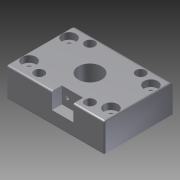
# Autodesk Inventor part: V5 Z Top bearing
Saved by Autodesk Inventor 2012 (Build 160160000, 160)
## iProperties
Created: 2013-02-06
Part Number: V5 Z Top bearing
Material: Default
Document SubType Name: Modeling
Designer: mce
Density: 1 g/cm^3
Mass: 38.3843 g
Surface Area: 115.42 cm^2
Volume: 38.3843 cm^3
Author: mce
Autodesk Inventor part; units mm, degrees
ref_plane "YZ Plane" through (0, 0, 0) normal (1, 0, 0) x (0, 1, 0)
ref_plane "XZ Plane" through (0, 0, 0) normal (0, 1, 0) x (-1, 0, 0)
ref_plane "XY Plane" through (0, 0, 0) normal (0, 0, 1) x (1, 0, 0)
sketch "Sketch1" plane through (0, 0, 0) normal (0, 0, 1) x (1, 0, 0)
  line L0 (0, 0) -> (60, 0)
  line L1 (60, 0) -> (60, 42.4)
  line L2 (60, 42.4) -> (0, 42.4)
  line L3 (0, 42.4) -> (0, 0)
  circle A0 centre (5, 33.4) radius 2.1
  circle A1 centre (55, 33.4) radius 2.1
  circle A2 centre (55, 9) radius 2.1
  circle A3 centre (5, 9) radius 2.1
  circle A4 centre (30, 21.2) radius 5
  circle A5 centre (14.5, 36.7) radius 3
  circle A6 centre (45.5, 36.7) radius 3
  circle A7 centre (45.5, 5.7) radius 3
  circle A8 centre (14.5, 5.7) radius 3
  dimension "d0" = 42.4
  dimension "d1" = 60
  dimension "d2" = 10
  dimension "d3" = 4.2
  dimension "d4" = 24.4
  dimension "d5" = 50
  dimension "d6" = 9
  dimension "d7" = 5
  dimension "d8" = 6
  dimension "d9" = 31
  dimension "d10" = 31
  dimension "d11" = 5.7
  dimension "d12" = 14.5
  dimension "d13" = 30
  dimension "d14" = 21.2
  constraints: 9 centre point, 8 end point, 6 equal radius, 4 horizontal alignment, 4 vertical alignment, 2 horizontal, 2 vertical
  measures "d0" distance of L2.end L0.start
  measures "d1" distance of L0.start L0.end
  measures "d2" diameter of A4
  measures "d3" diameter of A0
  measures "d4" distance of A3.centre A0.centre
  measures "d5" distance of A0.centre A1.centre
  measures "d6" distance from line of L2 A0.centre
  measures "d7" distance from line of L3 A0.centre
  measures "d8" diameter of A5
  measures "d9" distance of A6.centre A5.centre
  measures "d10" distance of A8.centre A5.centre
  measures "d11" distance from line of L0 A7.centre
  measures "d12" distance from line of L3 A8.centre
  measures "d13" distance from line of L3 A4.centre
  measures "d14" distance from line of L0 A4.centre
extrude "Extrusion1" add sketch "Sketch1" along normal blind 18
fillet "Fillet1" radius 1 11 edges at (0, 42.4, 9) (60, 42.4, 9) (30, 42.4, 0) (60, 21.2, 18) (30, 0, 18) (0, 21.2, 18) (0, 0, 9) (0, 21.2, 0) (60, 0, 9) (60, 21.2, 0) (30, 0, 0)
fillet "Fillet2" radius 3 3 edges at (30, 42.4, 18) (59.7071, 42.1071, 17.7071) (0.2929, 42.1071, 17.7071)
sketch "Sketch2" plane through (0, 0, 18) normal (0, 0, 1) x (1, 0, 0)
  circle A0 centre (5, 33.4) radius 2.1 projected
  circle A1 centre (55, 33.4) radius 2.1 projected
  circle A2 centre (55, 9) radius 2.1 projected
  circle A3 centre (5, 9) radius 2.1 projected
  circle A4 centre (5, 33.4) radius 4.25
  circle A5 centre (55, 33.4) radius 4.25
  circle A6 centre (55, 9) radius 4.25
  circle A7 centre (5, 9) radius 4.25
  point P0 (0, 0)
  dimension "d19" = 8.5
  constraints: 4 centre point, 4 coincident, 3 equal radius
  measures "d19" diameter of A4
extrude "Extrusion2" cut sketch "Sketch2" against normal blind 4
sketch "Sketch3" plane through (1, 0, 1) normal (0, -1, 0) x (1, 0, 0)
  line L0 (27, 17) -> (40, 17)
  line L1 (40, 17) -> (40, 7)
  line L2 (40, 7) -> (27, 7)
  line L3 (27, 7) -> (27, 17)
  line L4 (58, 17) -> (0, 17) projected
  line L5 (59, 0) -> (59, 16) projected
  point P0 (-1, -1)
  dimension "d22" = 19
  dimension "d23" = 13
  dimension "d24" = 10
  constraints: 8 end point, 1 collinear
  measures "d22" distance between parallel lines of L1 L5
  measures "d23" distance between parallel lines of L3 L1
  measures "d24" distance between parallel lines of L0 L2
extrude "Extrusion3" cut sketch "Sketch3" against normal blind 6
sketch "Sketch4" plane through (1, 0, 1) normal (0, -1, 0) x (1, 0, 0)
  line L0 (27, 7) -> (27, 16) projected
  circle A0 centre (30.25, 12) radius 1.05
  circle A1 centre (36.75, 12) radius 1.05
  line L1 (27, 17) -> (0, 17) projected
  point P0 (-1, -1)
  dimension "d27" = 2.1
  dimension "d28" = 5
  dimension "d29" = 6.5
  dimension "d30" = 3.25
  constraints: 2 centre point, 1 equal radius, 1 horizontal alignment
  measures "d27" diameter of A0
  measures "d28" distance from line of L1 A0.centre
  measures "d29" distance of A1.centre A0.centre
  measures "d30" distance from line of L0 A0.centre
extrude "Extrusion4" cut sketch "Sketch4" against normal blind 14
sketch "Sketch5" plane through (0, 0, 18) normal (0, 0, 1) x (1, 0, 0)
  circle A0 centre (30, 21.2) radius 5 projected
  circle A1 centre (30, 21.2) radius 7.1
  point P0 (0, 0)
  dimension "d33" = 14.2
  constraints: 1 centre point, 1 coincident
  measures "d33" diameter of A1
extrude "Extrusion5" cut sketch "Sketch5" against normal blind 15.5
equation "\"d6\" = -0.5 * d4 + 0.5 * d0"
equation "\"d7\" = -0.5 * d5 + 0.5 * d1"
equation "\"d11\" = -0.5 * d10 + 0.5 * d0"
equation "\"d12\" = -0.5 * d9 + 0.5 * d1"
equation "\"d13\" = 0.5 * d1"
equation "\"d14\" = 0.5 * d0"
body "Solid1"
